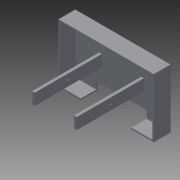
# Autodesk Inventor part: Base
Saved by Autodesk Inventor 2014 (Build 180170000, 170)
## iProperties
Created: 2014-01-05
Part Number: Base
Material: Generic
Document SubType Name: Modeling
Designer: Tristan Debrunner
Density: 1 g/cm^3
Appearance: Default
Author: Tristan Debrunner
Autodesk Inventor part; units mm, degrees
ref_plane "YZ Plane" through (0, 0, 0) normal (1, 0, 0) x (0, 1, 0)
ref_plane "XZ Plane" through (0, 0, 0) normal (0, 1, 0) x (-1, 0, 0)
ref_plane "XY Plane" through (0, 0, 0) normal (0, 0, 1) x (1, 0, 0)
sketch "Sketch1" plane through (0, 0, 0) normal (0, 0, 1) x (1, 0, 0)
  line L0 (-431.8, -266.7) -> (431.8, -266.7)
  line L1 (431.8, -266.7) -> (431.8, 266.7)
  line L2 (431.8, 266.7) -> (-431.8, 266.7)
  line L3 (-431.8, 266.7) -> (-431.8, -266.7)
  line L4 (-431.8, -266.7) -> (431.8, 266.7) construction
  line L5 (431.8, -266.7) -> (-431.8, 266.7) construction
  point P0 (0, 0)
  dimension "d0" = 863.6
  dimension "d1" = 533.4
  constraints: 12 end point, 2 midpoint, 2 parallel, 1 horizontal, 1 perpendicular
  measures "d0" distance of L2.end L1.end
  measures "d1" distance of L1.end L0.end
extrude "Extrusion1" add sketch "Sketch1" along normal blind 152.4
sketch "Sketch2" plane through (431.8, -266.7, 0) normal (1, 0, 0) x (0, 0, -1)
  line L0 (0, 0) -> (0, 533.4) projected
  line L1 (0, 0) -> (-152.4, 0) projected
  arc A0 (0, 387.7039) -> (0, 501.2961) centre (-50.8, 444.5) ccw
  line L2 (0, 266.7) -> (-335.0591, 266.7) construction
  line L3 (0, 501.2961) -> (0, 387.7039)
  arc A1 (0, 32.1039) -> (0, 145.6961) centre (-50.8, 88.9) ccw
  line L4 (0, 32.1039) -> (0, 145.6961)
  constraints: 6 end point, 4 point on circle, 3 symmetric about line, 2 centre point, 2 point on line, 1 collinear, 1 parallel, 1 other
extrude "Extrusion2" add sketch "Sketch2" against normal blind 76.2
extrude "Extrusion3" cut sketch "Sketch2" against normal blind 50.8
sketch "Sketch3" plane through (-431.8, -266.7, 0) normal (-1, 0, 0) x (0, 0, 1)
  line L0 (0, 501.2961) -> (0, 387.7039) projected
  arc A0 (0, 501.2961) -> (0, 387.7039) centre (50.8, 444.5) ccw projected
  line L1 (0, 145.6961) -> (0, 32.1039) projected
  arc A1 (0, 145.6961) -> (0, 32.1039) centre (50.8, 88.9) ccw projected
  point P0 (0, 266.7)
extrude "Extrusion4" add sketch "Sketch3" against normal blind 76.2
extrude "Extrusion5" cut sketch "Sketch3" against normal blind 50.8
sketch "Sketch4" plane through (0, 0, 152.4) normal (0, 0, 1) x (1, 0, 0)
  line L0 (-419.1, -254) -> (419.1, -254)
  line L1 (419.1, -254) -> (419.1, 254)
  line L2 (419.1, 254) -> (-419.1, 254)
  line L3 (-419.1, 254) -> (-419.1, -254)
  line L4 (-419.1, -254) -> (419.1, 254) construction
  line L5 (419.1, -254) -> (-419.1, 254) construction
  point P0 (0, 0)
  dimension "d14" = 838.2
  dimension "d15" = 508
  constraints: 12 end point, 2 midpoint, 2 parallel, 1 horizontal, 1 perpendicular
  measures "d14" distance of L2.end L1.end
  measures "d15" distance of L1.end L0.end
extrude "Extrusion6" cut sketch "Sketch4" against normal blind 139.7
sketch "Sketch5" plane through (0, 0, 12.7) normal (0, 0, 1) x (1, 0, 0)
  line L0 (203.2, -50.8) -> (177.8, -50.8)
  line L1 (177.8, -50.8) -> (177.8, 50.8)
  line L2 (177.8, 50.8) -> (203.2, 50.8)
  line L3 (203.2, 50.8) -> (203.2, -50.8)
  line L4 (203.2, -50.8) -> (177.8, 50.8) construction
  line L5 (177.8, -50.8) -> (203.2, 50.8) construction
  line L6 (-203.2, -50.8) -> (-177.8, -50.8)
  line L7 (-177.8, -50.8) -> (-177.8, 50.8)
  line L8 (-177.8, 50.8) -> (-203.2, 50.8)
  line L9 (-203.2, 50.8) -> (-203.2, -50.8)
  point P0 (0, 0)
  dimension "d19" = 25.4
  dimension "d20" = 101.6
  constraints: 20 end point, 2 parallel, 1 horizontal, 1 perpendicular
  measures "d19" distance of L1.end L2.end
  measures "d20" distance of L0.end L1.end
extrude "Extrusion7" add sketch "Sketch5" along normal blind 609.6
sketch "Sketch6" plane through (203.2, -50.8, 12.7) normal (1, 0, 0) x (0, 0, -1)
  line L0 (-609.6, 0) -> (-609.6, 101.6) projected
  line L1 (0, 0) -> (-609.6, 0) projected
  line L2 (-609.6, 50.8) -> (-304.8, 50.8)
  point P0 (12.7, 50.8)
  dimension "d23" = 304.8
  constraints: 2 end point, 1 midpoint, 1 parallel
  measures "d23" distance of L2.start L2.end
hole "Hole1" at (203.2, 0, 317.5) direction (-1, 0, 0) diameter 12.7 end through all
sketch "Sketch7" plane through (0, 0, 152.4) normal (0, 0, 1) x (1, 0, 0)
  line L0 (-431.8, -266.7) -> (431.8, -266.7) projected
  line L1 (0, -266.7) -> (228.6, -266.7)
  line L2 (228.6, -266.7) -> (228.6, -186.436)
  line L3 (228.6, -186.436) -> (-228.6, -186.436)
  line L4 (-228.6, -186.436) -> (-228.6, -266.7)
  line L5 (0, -266.7) -> (-228.6, -266.7)
  point P0 (0, 0)
  dimension "d31" = 228.6
  dimension "d32" = 80.264
  dimension "d33" = 457.2
  constraints: 10 end point, 3 perpendicular, 2 point on line, 1 collinear, 1 midpoint
  measures "d31" distance of L1.start L1.end
  measures "d32" distance of L1.end L2.end
  measures "d33" distance of L2.end L3.end
extrude "Extrusion8" cut sketch "Sketch7" against normal through all
body "Solid1"
